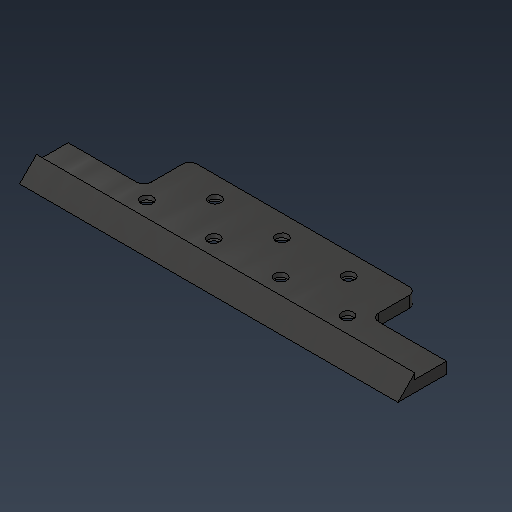
# Autodesk Inventor part: Plog2
Saved by Autodesk Inventor 2026.2 (Build 302298010, 298A)
## iProperties
Created: 2022-01-27
Part Number: Plog2
Material: Steel, Carbon
Document SubType Name: Modeling
Designer: Michał
Density: 7.85 g/cm^3
Appearance: Dark Gray
Mass: 42.0797 g
Surface Area: 48.5187 cm^2
Volume: 5.36047 cm^3
Author: Michał
Autodesk Inventor part; units mm, degrees
ref_plane "YZ Plane" through (0, 0, 0) normal (1, 0, 0) x (0, 1, 0)
ref_plane "XZ Plane" through (0, 0, 0) normal (0, 1, 0) x (-1, 0, 0)
ref_plane "XY Plane" through (0, 0, 0) normal (0, 0, 1) x (1, 0, 0)
sketch "Szkic1" plane through (0, 0, 0) normal (1, 0, 0) x (0, 1, 0)
  line L0 (0, 0) -> (3, -3)
  line L1 (3, -3) -> (3, -25)
  line L2 (3, -25) -> (0, -25)
  line L3 (0, -25) -> (0, -3)
  line L4 (0, -3) -> (0, 0)
  line L5 (0, -3) -> (3, -3)
  line L6 (3, -3) -> (4.5, -4.5)
  line L7 (4.5, -4.5) -> (3, -4.5)
  line L8 (3, -3) -> (4.5, -4.5)
  line L9 (4.5, -4.5) -> (3, -4.5)
  line L10 (4.5, -4.5) -> (4.5, -4.5)
  point P0 (5, -5)
  dimension "d1" = 3
  dimension "d2" = 45
  dimension "d44" = 45
  dimension "d45" = 3
  dimension "d46" = 22
  dimension "d50" = 4.5
  dimension "d51" = 25
  dimension "d54" = 0
  dimension "d98" = 1.5
  constraints: 22 end point, 6 perpendicular, 6 point on line, 1 vertical
  measures "d1" distance between parallel lines of L4 L1
  measures "d2" angle of L4 L0
  measures "d44" angle of L7 L6
  measures "d45" distance of L3.end L0.start
  measures "d46" distance of L2.end L3.end
  measures "d50" distance from line of L0.start L10
  measures "d51" distance from line of L2 L0.start
  measures "d54" distance from line of L10 L8.end
  measures "d98" distance from line of L1 L6.end
extrude "Wyciągnięcie proste1" add sketch "Szkic1" along normal mid plane 100
sketch "Sketch4" plane through (-50, 0, -25) normal (0, -1, 0) x (1, 0, 0)
  line L0 (0, 0) -> (0, 25) projected
  line L1 (0, 0) -> (100, 0) projected
  line L2 (100, 25) -> (100, 0) projected
  line L3 (100, 25) -> (0, 25) projected
  line L4 (80, 0) -> (80, 25)
  line L5 (100, 25) -> (50, 25) projected
  line L6 (20, 25) -> (20, 0)
  circle A0 centre (67.6667, 5.6667) radius 3.5
  circle A1 centre (50, 5.6667) radius 3.5
  circle A2 centre (32.3333, 5.6667) radius 3.5
  line L7 (0, 0) -> (100, 0) projected
  line L8 (0, 20.5) -> (100, 20.5) projected
  line L9 (80, 5.6667) -> (20, 5.6667)
  circle A3 centre (76.5, 14.8333) radius 3.5
  circle A4 centre (58.8333, 14.8333) radius 3.5
  circle A5 centre (41.1667, 14.8333) radius 3.5
  circle A6 centre (23.5, 14.8333) radius 3.5
  line L10 (80, 14.8333) -> (20, 14.8333)
  line L11 (76.5, 11.3333) -> (85, 11.3333) construction
  line L12 (85, 11.3333) -> (85, 9.1667) construction
  line L13 (85, 9.1667) -> (67.6667, 9.1667) construction
  line L14 (67.6667, 5.6667) -> (67.6667, 9.1667) construction
  line L15 (76.5, 11.3333) -> (76.5, 14.8333) construction
  line L16 (76.5, 14.8333) -> (76.5, 11.3333) construction
  dimension "d24" = 7
  dimension "d70" = 7
  dimension "d22" = 20
  dimension "d23" = 20
  dimension "d26" = 7
  dimension "d27" = 7
  dimension "d67" = 7
  dimension "d68" = 7
  dimension "d69" = 7
  dimension "d72" = 17.6667
  dimension "d75" = 17.6667
  dimension "d77" = 17.6667
  dimension "d82" = 8.8333
  dimension "d85" = 8.8333
  dimension "d86" = 8.8333
  dimension "d87" = 8.8333
  dimension "d88" = 8.8333
  dimension "d89" = 2.1667
  dimension "d90" = 2.1667
  dimension "d95" = 8.8333
  dimension "d96" = 2.1667
  dimension "d97" = 5
  constraints: 20 end point, 12 point on line, 5 centre point, 5 perpendicular, 3 horizontal, 2 point on circle, 2 vertical, 1 collinear, 1 horizontal alignment, 1 midpoint, 1 tangent, 1 vertical alignment, 4 other
  measures "d22" distance between parallel lines of L2 L4
  measures "d23" distance between parallel lines of L0 L6
  measures "d26" diameter of A1
  measures "d27" diameter of A2
  measures "d67" diameter of A3
  measures "d68" diameter of A4
  measures "d69" diameter of A5
  measures "d72" distance of A4.centre L15.end
  measures "d75" distance of point (23.5, 14.833) A5.centre
  measures "d77" distance of A5.centre A4.centre
  measures "d82" horizontal distance of A4.centre L14.start
  measures "d85" horizontal distance of A1.centre A4.centre
  measures "d86" horizontal distance of A1.centre A5.centre
  measures "d87" horizontal distance of A2.centre A5.centre
  measures "d88" horizontal distance of A2.centre point (23.5, 14.833)
  measures "d89" distance edge to line of A3 L8
  measures "d95" horizontal distance of L14.start L15.end
  measures "d96" distance of L11.end L12.end
  measures "d97" distance between parallel lines of L4 L12
hole "Hole2" at (17.6667, 0, -19.3333) at (0, 0, -19.3333) at (-17.6667, 0, -19.3333) at (26.5, 0, -10.1667) at (8.8333, 0, -10.1667) at (-8.8333, 0, -10.1667) at (-26.5, 0, -10.1667) direction (0, 1, 0) diameter 3.2 depth 8.8 countersink diameter 7 countersink angle 90 clearance for "Countersunk Flat Head Screw ISO 2009/7046" size "M3" standard "ISO"
sketch "Sketch5" plane through (-50, 0, 0) normal (0, -1, 0) x (1, 0, 0)
  line L0 (0, -25) -> (100, -25) projected
  circle A0 centre (32.3333, -19.3333) radius 3.5 projected
  circle A1 centre (50, -19.3333) radius 3.5 projected
  circle A2 centre (67.6667, -19.3333) radius 3.5 projected
  line L1 (100, 0) -> (100, -25) projected
  line L2 (100, 0) -> (0, 0) projected
  line L3 (0, -25) -> (0, 0) projected
  line L4 (100, -12.868) -> (80, -12.868)
  line L5 (80, -12.868) -> (80, -25)
  line L6 (80, -25) -> (100, -25)
  line L7 (100, -25) -> (100, -12.868)
  line L8 (0, -25) -> (20, -25)
  line L9 (20, -25) -> (20, -12.868)
  line L10 (20, -12.868) -> (0, -12.868)
  line L11 (0, -12.868) -> (0, -25)
  point P0 (50, 0)
  point P1 (0, -12.868)
  dimension "d55" = 20
  dimension "d56" = 20
  dimension "d61" = 12.868
  dimension "d62" = 12.868
  dimension "d65" = 0
  constraints: 16 end point, 4 parallel, 2 horizontal, 2 perpendicular, 1 point on line
  measures "d55" distance of L9.end L10.end
  measures "d56" distance of L4.start L4.end
  measures "d61" distance between parallel lines of L2 L10
  measures "d62" distance between parallel lines of L2 L4
  measures "d65" distance between parallel lines of L6 L0
extrude "Extrusion5" cut sketch "Sketch5" against normal through all contours L3 L10 L9 L0 | L5 L4 L1 L0
fillet "Fillet2" radius 2 4 edges at (30, 1.5, -12.868) (-30, 1.5, -12.868) (-30, 1.5, -25) (30, 1.5, -25)
equation "\"d23\" = d22"
equation "\"d72\" = d75"
equation "\"d77\" = d75"
equation "\"d56\" = d55"
equation "\"d62\" = d61"
equation "\"d64\" = d80"
equation "\"d79\" = d64"
equation "\"d80\" = 4.648267"
